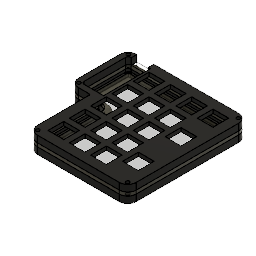
yampad_v2-Fusion360 (Autodesk Fusion 360 design; units mm, degrees)
Autodesk Fusion 360 part; units mm, degrees
(part 1 of 2)
sketch "PCB" plane through (0, 0, 0) normal (0, 1, 0) x (1, 0, 0) in component "MidLayer"
  line L0 (94.361, -93.472) -> (94.361, -1.778) construction
  arc A0 (-0.127, -38.608) -> (1.143, -39.878) centre (1.143, -38.608) ccw construction
  line L1 (92.583, 0) -> (1.397, 0) construction
  arc A1 (94.361, -1.778) -> (92.583, 0) centre (92.583, -1.778) ccw construction
  arc A2 (17.907, -93.218) -> (19.685, -94.996) centre (19.685, -93.218) ccw construction
  line L2 (17.907, -93.218) -> (17.907, -41.148) construction
  line L3 (19.685, -94.996) -> (92.837, -94.996) construction
  arc A3 (17.907, -41.148) -> (16.637, -39.878) centre (16.637, -41.148) ccw construction
  arc A4 (1.397, 0) -> (-0.127, -1.524) centre (1.397, -1.524) ccw construction
  line L4 (-0.127, -38.608) -> (-0.127, -1.524) construction
  arc A5 (92.837, -94.996) -> (94.361, -93.472) centre (92.837, -93.472) ccw construction
  line L5 (16.637, -39.878) -> (1.143, -39.878) construction
  line L6 (16.637, -39.878) -> (1.143, -39.878) construction
  line L7 (77.978, -44.958) -> (77.978, -30.988) construction
  line L8 (-0.127, -38.608) -> (-0.127, -1.524) construction
  arc A6 (92.837, -94.996) -> (94.361, -93.472) centre (92.837, -93.472) ccw construction
  arc A7 (94.361, -1.778) -> (92.583, 0) centre (92.583, -1.778) ccw construction
  line L9 (91.948, -30.988) -> (91.948, -44.958) construction
  line L10 (5.334, -3.81) -> (5.334, 1.524) construction
  line L11 (94.361, -93.472) -> (94.361, -1.778) construction
  line L12 (39.878, -16.383) -> (39.878, -2.413) construction
  line L13 (12.954, 1.524) -> (12.954, -3.81) construction
  line L14 (58.928, -2.413) -> (72.898, -2.413) construction
  line L15 (91.948, -44.958) -> (77.978, -44.958) construction
  line L16 (72.898, -40.513) -> (72.898, -54.483) construction
  line L17 (77.978, -2.413) -> (91.948, -2.413) construction
  line L18 (77.978, -69.088) -> (91.948, -69.088) construction
  line L19 (58.928, -21.463) -> (72.898, -21.463) construction
  line L20 (39.878, -21.463) -> (53.848, -21.463) construction
  line L21 (72.898, -21.463) -> (72.898, -35.433) construction
  line L22 (17.907, -93.218) -> (17.907, -41.148) construction
  arc A8 (1.397, 0) -> (-0.127, -1.524) centre (1.397, -1.524) ccw construction
  arc A9 (17.907, -41.148) -> (16.637, -39.878) centre (16.637, -41.148) ccw construction
  line L23 (12.954, -3.81) -> (5.334, -3.81) construction
  line L24 (39.878, -2.413) -> (53.848, -2.413) construction
  line L25 (72.898, -35.433) -> (58.928, -35.433) construction
  line L26 (39.878, -35.433) -> (39.878, -21.463) construction
  line L27 (58.928, -16.383) -> (58.928, -2.413) construction
  line L28 (72.898, -16.383) -> (58.928, -16.383) construction
  line L29 (20.828, -40.513) -> (34.798, -40.513) construction
  line L30 (91.948, -2.413) -> (91.948, -16.383) construction
  line L31 (91.948, -16.383) -> (77.978, -16.383) construction
  line L32 (53.848, -21.463) -> (53.848, -35.433) construction
  line L33 (77.978, -83.058) -> (77.978, -69.088) construction
  line L34 (53.848, -16.383) -> (39.878, -16.383) construction
  line L35 (72.898, -54.483) -> (58.928, -54.483) construction
  line L36 (58.928, -40.513) -> (72.898, -40.513) construction
  line L37 (77.978, -30.988) -> (91.948, -30.988) construction
  line L38 (91.948, -83.058) -> (77.978, -83.058) construction
  arc A10 (-0.127, -38.608) -> (1.143, -39.878) centre (1.143, -38.608) ccw construction
  line L39 (0, -39.878) -> (0, 0) construction
  arc A11 (17.907, -93.218) -> (19.685, -94.996) centre (19.685, -93.218) ccw construction
  line L40 (91.948, -69.088) -> (91.948, -83.058) construction
  line L41 (0, 0) -> (18.161, 0) construction
  line L42 (18.161, -39.878) -> (0, -39.878) construction
  line L43 (5.334, 1.524) -> (12.954, 1.524) construction
  line L44 (18.161, 0) -> (18.161, -39.878) construction
  line L45 (20.828, -35.433) -> (20.828, -21.463) construction
  line L46 (92.583, 0) -> (1.397, 0) construction
  line L47 (19.685, -94.996) -> (92.837, -94.996) construction
  line L48 (34.798, -35.433) -> (20.828, -35.433) construction
  line L49 (72.898, -59.563) -> (72.898, -73.533) construction
  line L50 (34.798, -73.533) -> (20.828, -73.533) construction
  line L51 (34.798, -92.583) -> (20.828, -92.583) construction
  line L52 (39.878, -54.483) -> (39.878, -40.513) construction
  line L53 (53.848, -78.613) -> (53.848, -92.583) construction
  line L54 (58.928, -73.533) -> (58.928, -59.563) construction
  line L55 (39.878, -78.613) -> (53.848, -78.613) construction
  line L56 (53.848, -92.583) -> (39.878, -92.583) construction
  line L57 (20.828, -21.463) -> (34.798, -21.463) construction
  line L58 (34.798, -78.613) -> (34.798, -92.583) construction
  line L59 (58.928, -59.563) -> (72.898, -59.563) construction
  line L60 (34.798, -21.463) -> (34.798, -35.433) construction
  line L61 (34.798, -16.383) -> (20.828, -16.383) construction
  line L62 (53.848, -59.563) -> (53.848, -73.533) construction
  line L63 (20.828, -54.483) -> (20.828, -40.513) construction
  line L64 (39.878, -40.513) -> (53.848, -40.513) construction
  line L65 (39.878, -73.533) -> (39.878, -59.563) construction
  line L66 (53.848, -73.533) -> (39.878, -73.533) construction
  line L67 (53.848, -40.513) -> (53.848, -54.483) construction
  line L68 (72.898, -73.533) -> (58.928, -73.533) construction
  line L69 (20.828, -78.613) -> (34.798, -78.613) construction
  line L70 (58.928, -35.433) -> (58.928, -21.463) construction
  line L71 (39.878, -92.583) -> (39.878, -78.613) construction
  line L72 (20.828, -92.583) -> (20.828, -78.613) construction
  line L73 (34.798, -59.563) -> (34.798, -73.533) construction
  line L74 (58.928, -92.583) -> (58.928, -78.613) construction
  line L75 (53.848, -54.483) -> (39.878, -54.483) construction
  line L76 (77.978, -16.383) -> (77.978, -2.413) construction
  line L77 (72.898, -92.583) -> (58.928, -92.583) construction
  line L78 (20.828, -59.563) -> (34.798, -59.563) construction
  line L79 (58.928, -78.613) -> (72.898, -78.613) construction
  line L80 (20.828, -16.383) -> (20.828, -2.413) construction
  line L81 (20.828, -73.533) -> (20.828, -59.563) construction
  line L82 (53.848, -35.433) -> (39.878, -35.433) construction
  line L83 (58.928, -54.483) -> (58.928, -40.513) construction
  line L84 (53.848, -2.413) -> (53.848, -16.383) construction
  line L85 (72.898, -78.613) -> (72.898, -92.583) construction
  line L86 (34.798, -2.413) -> (34.798, -16.383) construction
  line L87 (34.798, -54.483) -> (20.828, -54.483) construction
  line L88 (34.798, -40.513) -> (34.798, -54.483) construction
  line L89 (20.828, -2.413) -> (34.798, -2.413) construction
  line L90 (39.878, -59.563) -> (53.848, -59.563) construction
  line L91 (72.898, -2.413) -> (72.898, -16.383) construction
  line L92 (95.361, -93.472) -> (95.361, -1.778)
  arc A12 (95.361, -1.778) -> (92.583, 1) centre (92.583, -1.778) ccw
  line L93 (92.583, 1) -> (1.397, 1)
  arc A13 (1.397, 1) -> (-1.127, -1.524) centre (1.397, -1.524) ccw
  line L94 (-1.127, -38.608) -> (-1.127, -1.524)
  arc A14 (-1.127, -38.608) -> (1.143, -40.878) centre (1.143, -38.608) ccw
  line L95 (16.637, -40.878) -> (1.143, -40.878) construction
  arc A15 (16.907, -41.148) -> (16.637, -40.878) centre (16.637, -41.148) ccw construction
  line L96 (16.907, -93.218) -> (16.907, -41.148) construction
  arc A16 (16.907, -93.218) -> (19.685, -95.996) centre (19.685, -93.218) ccw
  line L97 (19.685, -95.996) -> (92.837, -95.996)
  arc A17 (92.837, -95.996) -> (95.361, -93.472) centre (92.837, -93.472) ccw
  line L98 (100.361, -93.472) -> (100.361, -1.778)
  arc A18 (100.361, -1.778) -> (92.583, 6) centre (92.583, -1.778) ccw
  line L99 (92.583, 6) -> (1.397, 6)
  arc A19 (1.397, 6) -> (-6.127, -1.524) centre (1.397, -1.524) ccw
  line L100 (-6.127, -38.608) -> (-6.127, -1.524)
  arc A20 (-6.127, -38.608) -> (1.143, -45.878) centre (1.143, -38.608) ccw
  line L101 (11.907, -45.878) -> (1.143, -45.878) construction
  line L102 (11.907, -93.218) -> (11.907, -45.878) construction
  arc A21 (11.907, -93.218) -> (19.685, -100.996) centre (19.685, -93.218) ccw
  line L103 (19.685, -100.996) -> (92.837, -100.996)
  arc A22 (92.837, -100.996) -> (100.361, -93.472) centre (92.837, -93.472) ccw
  line L104 (1.143, -40.878) -> (13.907, -40.878)
  line L105 (16.907, -93.218) -> (16.907, -43.878)
  arc A23 (16.907, -43.878) -> (13.907, -40.878) centre (13.907, -43.878) ccw
  line L106 (1.143, -45.878) -> (10.907, -45.878)
  line L107 (11.907, -46.878) -> (11.907, -93.218)
  arc A24 (11.907, -46.878) -> (10.907, -45.878) centre (10.907, -46.878) ccw
  dimension "d7" = 1
  dimension "d8" = 6
  dimension "d10" = 3
  dimension "d11" = 1
  constraint tangent A14 L104
  constraint perpendicular L96 L104
  constraint tangent A16 L105
  constraint tangent L104 A23
  constraint tangent L105 A23
  constraint tangent A20 L106
  constraint tangent A21 L107
  constraint coincident L101.start L107
  constraint coincident L101.start L106
  constraint tangent L107 A24
  constraint tangent L106 A24
  measures "d10" radius of A23
  measures "d11" radius of A24
extrude "Extrude1" add sketch "PCB" along normal blind 3 makes body 1 in component "MidLayer"
sketch "Sketch1" plane through (0, 3, 0) normal (0, 1, 0) x (-1, 0, 0) in component "TopLayer"
  arc A0 (-16.907, 93.218) -> (-19.685, 95.996) centre (-19.685, 93.218) ccw construction
  line L0 (-16.907, 93.218) -> (-16.907, 43.878) construction
  arc A1 (-16.907, 43.878) -> (-13.907, 40.878) centre (-13.907, 43.878) ccw construction
  line L1 (-13.907, 40.878) -> (-1.143, 40.878)
  arc A2 (1.127, 38.608) -> (-1.143, 40.878) centre (-1.143, 38.608) ccw
  line L2 (1.127, 38.608) -> (1.127, 1.524)
  arc A3 (-1.397, -1) -> (1.127, 1.524) centre (-1.397, 1.524) ccw
  line L3 (-1.397, -1) -> (-92.583, -1) construction
  arc A4 (-95.361, 1.778) -> (-92.583, -1) centre (-92.583, 1.778) ccw construction
  line L4 (-95.361, 1.778) -> (-95.361, 93.472) construction
  arc A5 (-92.837, 95.996) -> (-95.361, 93.472) centre (-92.837, 93.472) ccw construction
  line L5 (-92.837, 95.996) -> (-19.685, 95.996) construction
  arc A6 (-11.907, 93.218) -> (-19.685, 100.996) centre (-19.685, 93.218) ccw
  line L6 (-19.685, 100.996) -> (-92.837, 100.996)
  arc A7 (-92.837, 100.996) -> (-100.361, 93.472) centre (-92.837, 93.472) ccw
  line L7 (-100.361, 93.472) -> (-100.361, 1.778)
  arc A8 (-100.361, 1.778) -> (-92.583, -6) centre (-92.583, 1.778) ccw
  line L8 (-92.583, -6) -> (-1.397, -6)
  arc A9 (-1.397, -6) -> (6.127, 1.524) centre (-1.397, 1.524) ccw
  line L9 (6.127, 1.524) -> (6.127, 38.608)
  arc A10 (6.127, 38.608) -> (-1.143, 45.878) centre (-1.143, 38.608) ccw
  line L10 (-1.143, 45.878) -> (-10.907, 45.878)
  arc A11 (-11.907, 46.878) -> (-10.907, 45.878) centre (-10.907, 46.878) ccw
  line L11 (-11.907, 46.878) -> (-11.907, 93.218)
  line L12 (-20.828, 2.413) -> (-34.798, 16.383) construction
  line L13 (-39.878, 2.413) -> (-53.848, 16.383) construction
  line L14 (-58.928, 2.413) -> (-72.898, 16.383) construction
  line L15 (-77.978, 2.413) -> (-91.948, 16.383) construction
  line L16 (-20.828, 21.463) -> (-34.798, 35.433) construction
  line L17 (-39.878, 21.463) -> (-53.848, 35.433) construction
  line L18 (-58.928, 21.463) -> (-72.898, 35.433) construction
  line L19 (-77.978, 30.988) -> (-91.948, 44.958) construction
  line L20 (-20.828, 40.513) -> (-34.798, 54.483) construction
  line L21 (-39.878, 40.513) -> (-53.848, 54.483) construction
  line L22 (-58.928, 40.513) -> (-72.898, 54.483) construction
  line L23 (-20.828, 59.563) -> (-34.798, 73.533) construction
  line L24 (-39.878, 59.563) -> (-53.848, 73.533) construction
  line L25 (-58.928, 59.563) -> (-72.898, 73.533) construction
  line L26 (-77.978, 69.088) -> (-91.948, 83.058) construction
  line L27 (-20.828, 78.613) -> (-34.798, 92.583) construction
  line L28 (-39.878, 78.613) -> (-53.848, 92.583) construction
  line L29 (-58.928, 78.613) -> (-72.898, 92.583) construction
  line L30 (-34.838, 16.423) -> (-20.788, 16.423)
  line L31 (-20.788, 16.423) -> (-20.788, 2.373)
  line L32 (-20.788, 2.373) -> (-34.838, 2.373)
  line L33 (-34.838, 2.373) -> (-34.838, 16.423)
  line L34 (-34.838, 16.423) -> (-20.788, 2.373) construction
  line L35 (-20.788, 16.423) -> (-34.838, 2.373) construction
  line L36 (-53.888, 16.423) -> (-39.838, 16.423)
  line L37 (-39.838, 16.423) -> (-39.838, 2.373)
  line L38 (-39.838, 2.373) -> (-53.888, 2.373)
  line L39 (-53.888, 2.373) -> (-53.888, 16.423)
  line L40 (-53.888, 16.423) -> (-39.838, 2.373) construction
  line L41 (-39.838, 16.423) -> (-53.888, 2.373) construction
  line L42 (-34.838, 35.473) -> (-20.788, 35.473)
  line L43 (-20.788, 35.473) -> (-20.788, 21.423)
  line L44 (-20.788, 21.423) -> (-34.838, 21.423)
  line L45 (-34.838, 21.423) -> (-34.838, 35.473)
  line L46 (-34.838, 35.473) -> (-20.788, 21.423) construction
  line L47 (-20.788, 35.473) -> (-34.838, 21.423) construction
  line L48 (-72.938, 16.423) -> (-58.888, 16.423)
  line L49 (-58.888, 16.423) -> (-58.888, 2.373)
  line L50 (-58.888, 2.373) -> (-72.938, 2.373)
  line L51 (-72.938, 2.373) -> (-72.938, 16.423)
  line L52 (-72.938, 16.423) -> (-58.888, 2.373) construction
  line L53 (-58.888, 16.423) -> (-72.938, 2.373) construction
  line L54 (-91.988, 16.423) -> (-77.938, 16.423)
  line L55 (-77.938, 16.423) -> (-77.938, 2.373)
  line L56 (-77.938, 2.373) -> (-91.988, 2.373)
  line L57 (-91.988, 2.373) -> (-91.988, 16.423)
  line L58 (-91.988, 16.423) -> (-77.938, 2.373) construction
  line L59 (-77.938, 16.423) -> (-91.988, 2.373) construction
  line L60 (-53.888, 35.473) -> (-39.838, 35.473)
  line L61 (-39.838, 35.473) -> (-39.838, 21.423)
  line L62 (-39.838, 21.423) -> (-53.888, 21.423)
  line L63 (-53.888, 21.423) -> (-53.888, 35.473)
  line L64 (-53.888, 35.473) -> (-39.838, 21.423) construction
  line L65 (-39.838, 35.473) -> (-53.888, 21.423) construction
  line L66 (-72.938, 35.473) -> (-58.888, 35.473)
  line L67 (-58.888, 35.473) -> (-58.888, 21.423)
  line L68 (-58.888, 21.423) -> (-72.938, 21.423)
  line L69 (-72.938, 21.423) -> (-72.938, 35.473)
  line L70 (-72.938, 35.473) -> (-58.888, 21.423) construction
  line L71 (-58.888, 35.473) -> (-72.938, 21.423) construction
  line L72 (-91.988, 44.998) -> (-77.938, 44.998)
  line L73 (-77.938, 44.998) -> (-77.938, 30.948)
  line L74 (-77.938, 30.948) -> (-91.988, 30.948)
  line L75 (-91.988, 30.948) -> (-91.988, 44.998)
  line L76 (-91.988, 44.998) -> (-77.938, 30.948) construction
  line L77 (-77.938, 44.998) -> (-91.988, 30.948) construction
  line L78 (-72.938, 54.523) -> (-58.888, 54.523)
  line L79 (-58.888, 54.523) -> (-58.888, 40.473)
  line L80 (-58.888, 40.473) -> (-72.938, 40.473)
  line L81 (-72.938, 40.473) -> (-72.938, 54.523)
  line L82 (-72.938, 54.523) -> (-58.888, 40.473) construction
  line L83 (-58.888, 54.523) -> (-72.938, 40.473) construction
  line L84 (-53.888, 54.523) -> (-39.838, 54.523)
  line L85 (-39.838, 54.523) -> (-39.838, 40.473)
  line L86 (-39.838, 40.473) -> (-53.888, 40.473)
  line L87 (-53.888, 40.473) -> (-53.888, 54.523)
  line L88 (-53.888, 54.523) -> (-39.838, 40.473) construction
  line L89 (-39.838, 54.523) -> (-53.888, 40.473) construction
  line L90 (-34.838, 54.523) -> (-20.788, 54.523)
  line L91 (-20.788, 54.523) -> (-20.788, 40.473)
  line L92 (-20.788, 40.473) -> (-34.838, 40.473)
  line L93 (-34.838, 40.473) -> (-34.838, 54.523)
  line L94 (-34.838, 54.523) -> (-20.788, 40.473) construction
  line L95 (-20.788, 54.523) -> (-34.838, 40.473) construction
  line L96 (-34.838, 73.573) -> (-20.788, 73.573)
  line L97 (-20.788, 73.573) -> (-20.788, 59.523)
  line L98 (-20.788, 59.523) -> (-34.838, 59.523)
  line L99 (-34.838, 59.523) -> (-34.838, 73.573)
  line L100 (-34.838, 73.573) -> (-20.788, 59.523) construction
  line L101 (-20.788, 73.573) -> (-34.838, 59.523) construction
  line L102 (-53.888, 73.573) -> (-39.838, 73.573)
  line L103 (-39.838, 73.573) -> (-39.838, 59.523)
  line L104 (-39.838, 59.523) -> (-53.888, 59.523)
  line L105 (-53.888, 59.523) -> (-53.888, 73.573)
  line L106 (-53.888, 73.573) -> (-39.838, 59.523) construction
  line L107 (-39.838, 73.573) -> (-53.888, 59.523) construction
  line L108 (-72.938, 73.573) -> (-58.888, 73.573)
  line L109 (-58.888, 73.573) -> (-58.888, 59.523)
  line L110 (-58.888, 59.523) -> (-72.938, 59.523)
  line L111 (-72.938, 59.523) -> (-72.938, 73.573)
  line L112 (-72.938, 73.573) -> (-58.888, 59.523) construction
  line L113 (-58.888, 73.573) -> (-72.938, 59.523) construction
  line L114 (-91.988, 83.098) -> (-77.938, 83.098)
  line L115 (-77.938, 83.098) -> (-77.938, 69.048)
  line L116 (-77.938, 69.048) -> (-91.988, 69.048)
  line L117 (-91.988, 69.048) -> (-91.988, 83.098)
  line L118 (-91.988, 83.098) -> (-77.938, 69.048) construction
  line L119 (-77.938, 83.098) -> (-91.988, 69.048) construction
  line L120 (-72.938, 92.623) -> (-58.888, 92.623)
  line L121 (-58.888, 92.623) -> (-58.888, 78.573)
  line L122 (-58.888, 78.573) -> (-72.938, 78.573)
  line L123 (-72.938, 78.573) -> (-72.938, 92.623)
  line L124 (-72.938, 92.623) -> (-58.888, 78.573) construction
  line L125 (-58.888, 92.623) -> (-72.938, 78.573) construction
  line L126 (-53.888, 92.623) -> (-39.838, 92.623)
  line L127 (-39.838, 92.623) -> (-39.838, 78.573)
  line L128 (-39.838, 78.573) -> (-53.888, 78.573)
  line L129 (-53.888, 78.573) -> (-53.888, 92.623)
  line L130 (-53.888, 92.623) -> (-39.838, 78.573) construction
  line L131 (-39.838, 92.623) -> (-53.888, 78.573) construction
  line L132 (-34.838, 92.623) -> (-20.788, 92.623)
  line L133 (-20.788, 92.623) -> (-20.788, 78.573)
  line L134 (-20.788, 78.573) -> (-34.838, 78.573)
  line L135 (-34.838, 78.573) -> (-34.838, 92.623)
  line L136 (-34.838, 92.623) -> (-20.788, 78.573) construction
  line L137 (-20.788, 92.623) -> (-34.838, 78.573) construction
  line L138 (-18.161, 0) -> (0, 0) construction
  line L139 (0, 0) -> (0, 39.878) construction
  line L140 (0, 39.878) -> (-18.161, 39.878) construction
  line L141 (-18.161, 39.878) -> (-18.161, 0) construction
  line L142 (-16.644, -6) -> (-1.644, -6)
  line L143 (0.5, -0.5) -> (0.5, 40.378) construction
  line L144 (0.5, 40.378) -> (-18.661, 40.378) construction
  line L145 (-18.661, 40.378) -> (-18.661, -0.5)
  line L146 (-18.661, -0.5) -> (0.5, -0.5) construction
  line L147 (-18.661, -0.5) -> (-18.661, -1)
  line L148 (-18.661, -1) -> (-1.397, -1)
  line L149 (-13.907, 40.878) -> (-18.661, 40.878)
  line L150 (-18.661, 40.878) -> (-18.661, 40.378)
  line L151 (-12.954, -0.5) -> (-12.954, -6) construction
  line L152 (-92.583, -6) -> (-1.397, -6)
  line L153 (-12.954, -6) -> (-5.334, -0.5) construction
  line L154 (-1.644, -6) -> (-16.644, -6)
  line L155 (-16.644, -6) -> (-16.644, -0.5)
  line L156 (-16.644, -0.5) -> (-1.644, -0.5)
  line L157 (-1.644, -0.5) -> (-1.644, -6)
  line L158 (-1.644, -6) -> (-16.644, -0.5) construction
  line L159 (-16.644, -6) -> (-1.644, -0.5) construction
  point P0 (-20.828, 2.413)
  point P1 (-34.798, 16.383)
  point P2 (-39.878, 2.413)
  point P3 (-53.848, 16.383)
  point P4 (-58.928, 2.413)
  point P5 (-72.898, 16.383)
  point P6 (-77.978, 2.413)
  point P7 (-91.948, 16.383)
  point P8 (-20.828, 21.463)
  point P9 (-34.798, 35.433)
  point P10 (-39.878, 21.463)
  point P11 (-53.848, 35.433)
  point P12 (-58.928, 21.463)
  point P13 (-72.898, 35.433)
  point P14 (-77.978, 30.988)
  point P15 (-91.948, 44.958)
  point P16 (-20.828, 40.513)
  point P17 (-34.798, 54.483)
  point P18 (-39.878, 40.513)
  point P19 (-53.848, 54.483)
  point P20 (-58.928, 40.513)
  point P21 (-72.898, 54.483)
  point P22 (-20.828, 59.563)
  point P23 (-34.798, 73.533)
  point P24 (-39.878, 59.563)
  point P25 (-53.848, 73.533)
  point P26 (-58.928, 59.563)
  point P27 (-72.898, 73.533)
  point P28 (-77.978, 69.088)
  point P29 (-91.948, 83.058)
  point P30 (-20.828, 78.613)
  point P31 (-34.798, 92.583)
  point P32 (-39.878, 78.613)
  point P33 (-53.848, 92.583)
  point P34 (-58.928, 78.613)
  point P35 (-72.898, 92.583)
  point P36 (-27.813, 9.398)
  point P37 (-46.863, 9.398)
  point P38 (-27.813, 28.448)
  point P39 (-65.913, 9.398)
  point P40 (-84.963, 9.398)
  point P41 (-46.863, 28.448)
  point P42 (-65.913, 28.448)
  point P43 (-84.963, 37.973)
  point P44 (-65.913, 47.498)
  point P45 (-46.863, 47.498)
  point P46 (-27.813, 47.498)
  point P47 (-27.813, 66.548)
  point P48 (-46.863, 66.548)
  point P49 (-65.913, 66.548)
  point P50 (-84.963, 76.073)
  point P51 (-65.913, 85.598)
  point P52 (-46.863, 85.598)
  point P53 (-27.813, 85.598)
  point P54 (-18.161, 0)
  point P55 (0, 39.878)
  point P56 (-5.334, -0.5)
  point P57 (-12.954, -0.5)
  point P58 (-9.144, -3.25)
  dimension "d14" = 14.05
  dimension "d15" = 14.05
  dimension "d16" = 14.05
  dimension "d17" = 14.05
  dimension "d18" = 14.05
  dimension "d19" = 14.05
  dimension "d20" = 14.05
  dimension "d21" = 14.05
  dimension "d26" = 0.5
  dimension "d27" = 15
  constraint coincident P0 L12.start
  constraint coincident P1 L12.end
  constraint coincident P2 L13.start
  constraint coincident P3 L13.end
  constraint coincident P4 L14.start
  constraint coincident P5 L14.end
  constraint coincident P6 L15.start
  constraint coincident P7 L15.end
  constraint coincident P8 L16.start
  constraint coincident P9 L16.end
  constraint coincident P10 L17.start
  constraint coincident P11 L17.end
  constraint coincident P12 L18.start
  constraint coincident P13 L18.end
  constraint coincident P14 L19.start
  constraint coincident P15 L19.end
  constraint coincident P16 L20.start
  constraint coincident P17 L20.end
  constraint coincident P18 L21.start
  constraint coincident P19 L21.end
  constraint coincident P20 L22.start
  constraint coincident P21 L22.end
  constraint coincident P22 L23.start
  constraint coincident P23 L23.end
  constraint coincident P24 L24.start
  constraint coincident P25 L24.end
  constraint coincident P26 L25.start
  constraint coincident P27 L25.end
  constraint coincident P28 L26.start
  constraint coincident P29 L26.end
  constraint coincident P30 L27.start
  constraint coincident P31 L27.end
  constraint coincident P32 L28.start
  constraint coincident P33 L28.end
  constraint coincident P34 L29.start
  constraint coincident P35 L29.end
  constraint perpendicular L30 L31
  constraint parallel L30 L32
  constraint parallel L31 L33
  constraint horizontal L30
  constraint coincident L34 P36
  constraint coincident L35 P36
  constraint midpoint L12 P36
  constraint perpendicular L36 L37
  constraint parallel L36 L38
  constraint parallel L37 L39
  constraint horizontal L36
  constraint coincident L40 P37
  constraint coincident L41 P37
  constraint midpoint L13 P37
  constraint perpendicular L42 L43
  constraint parallel L42 L44
  constraint parallel L43 L45
  constraint horizontal L42
  constraint coincident L46 P38
  constraint coincident L47 P38
  constraint midpoint L16 P38
  constraint perpendicular L48 L49
  constraint parallel L48 L50
  constraint parallel L49 L51
  constraint horizontal L48
  constraint coincident L52 P39
  constraint coincident L53 P39
  constraint midpoint L14 P39
  constraint perpendicular L54 L55
  constraint parallel L54 L56
  constraint parallel L55 L57
  constraint horizontal L54
  constraint coincident L15 L54.start
  constraint coincident L58 P40
  constraint coincident L59 P40
  constraint midpoint L15 P40
  constraint equal L50 L56
  constraint perpendicular L60 L61
  constraint parallel L60 L62
  constraint parallel L61 L63
  constraint horizontal L60
  constraint coincident L17 L60.start
  constraint coincident L64 P41
  constraint coincident L65 P41
  constraint midpoint L17 P41
  constraint perpendicular L66 L67
  constraint parallel L66 L68
  constraint parallel L67 L69
  constraint horizontal L66
  constraint coincident L18 L66.start
  constraint coincident L70 P42
  constraint coincident L71 P42
  constraint midpoint L18 P42
  constraint perpendicular L72 L73
  constraint parallel L72 L74
  constraint parallel L73 L75
  constraint horizontal L72
  constraint coincident L19 L72.start
  constraint coincident L76 P43
  constraint coincident L77 P43
  constraint midpoint L19 P43
  constraint perpendicular L78 L79
  constraint parallel L78 L80
  constraint parallel L79 L81
  constraint horizontal L78
  constraint coincident L22 L78.start
  constraint coincident L82 P44
  constraint coincident L83 P44
  constraint midpoint L22 P44
  constraint perpendicular L84 L85
  constraint parallel L84 L86
  constraint parallel L85 L87
  constraint horizontal L84
  constraint coincident L21 L84.start
  constraint coincident L88 P45
  constraint coincident L89 P45
  constraint midpoint L21 P45
  constraint perpendicular L90 L91
  constraint parallel L90 L92
  constraint parallel L91 L93
  constraint horizontal L90
  constraint coincident L20 L90.start
  constraint coincident L94 P46
  constraint coincident L95 P46
  constraint midpoint L20 P46
  constraint equal L86 L92
  constraint equal L80 L86
  constraint equal L74 L80
  constraint equal L68 L74
  constraint equal L62 L68
  constraint equal L44 L62
  constraint perpendicular L96 L97
  constraint parallel L96 L98
  constraint parallel L97 L99
  constraint horizontal L96
  constraint coincident L23 L96.start
  constraint coincident L100 P47
  constraint coincident L101 P47
  constraint midpoint L23 P47
  constraint perpendicular L102 L103
  constraint parallel L102 L104
  constraint parallel L103 L105
  constraint horizontal L102
  constraint coincident L24 L102.start
  constraint coincident L106 P48
  constraint coincident L107 P48
  constraint midpoint L24 P48
  constraint perpendicular L108 L109
  constraint parallel L108 L110
  constraint parallel L109 L111
  constraint horizontal L108
  constraint coincident L25 L108.start
  constraint coincident L112 P49
  constraint coincident L113 P49
  constraint midpoint L25 P49
  constraint perpendicular L114 L115
  constraint parallel L114 L116
  constraint parallel L115 L117
  constraint horizontal L114
  constraint coincident L26 L114.start
  constraint coincident L118 P50
  constraint coincident L119 P50
  constraint midpoint L26 P50
  constraint perpendicular L120 L121
  constraint parallel L120 L122
  constraint parallel L121 L123
  constraint horizontal L120
  constraint coincident L29 L120.start
  constraint coincident L124 P51
  constraint coincident L125 P51
  constraint midpoint L29 P51
  constraint perpendicular L126 L127
  constraint parallel L126 L128
  constraint parallel L127 L129
  constraint horizontal L126
  constraint coincident L28 L126.start
  constraint coincident L130 P52
  constraint coincident L131 P52
  constraint midpoint L28 P52
  constraint perpendicular L132 L133
  constraint parallel L132 L134
  constraint parallel L133 L135
  constraint horizontal L132
  constraint coincident L27 L132.start
  constraint coincident L136 P53
  constraint coincident L137 P53
  constraint midpoint L27 P53
  constraint equal L98 L104
  constraint equal L104 L110
  constraint equal L110 L116
  constraint equal L116 L122
  constraint equal L122 L128
  constraint equal L128 L134
  constraint equal L72 L134
  constraint horizontal L138
  constraint vertical L139
  constraint horizontal L140
  constraint vertical L141
  constraint coincident P55 L139.end
  constraint coincident P54 L138.start
  constraint horizontal L142
  constraint coincident L3 L147.end
  constraint perpendicular L3 L147
  constraint coincident A3.start L3.start
  constraint coincident A1.end L1.start
  constraint tangent A1 L149
  constraint perpendicular L145 L149
  constraint perpendicular L144 L150
  constraint coincident P57 L151.start
  constraint perpendicular L146 L151
  constraint coincident L151.end L152
  constraint coincident P56 L153.end
  constraint perpendicular L154 L155
  constraint parallel L154 L156
  constraint parallel L155 L157
  constraint horizontal L154
  constraint coincident L158 P58
  constraint coincident L159 P58
  constraint midpoint L153 P58
  measures "d14" distance of L31.end L32.end
  measures "d15" distance of L30.end L31.end
  measures "d16" distance of L37.end L38.end
  measures "d17" distance of L36.end L37.end
  measures "d18" distance of L43.end L44.end
  measures "d19" distance of L42.end L43.end
  measures "d20" distance of L48.end L49.end
  measures "d21" distance of L49.end L50.end
  measures "d27" distance of L155.end L156.end
extrude "Extrude1'" add sketch "Sketch1" along normal blind 6 separate body contours L1 A2 L2 A3 A6 L6 A7 L7 A8 L8 A9 L9 A10 L10 A11 L11 L145 L147 L148 L149 L150 L152 L155 L157 makes body 2 in component "TopLayer"
sketch "Sketch2" plane through (0, 3, 0) normal (0, -1, 0) x (1, 0, 0) in component "TopLayer"
  line L0 (91.988, 2.373) -> (77.938, 2.373)
  line L1 (77.938, 2.373) -> (77.938, 16.423)
  line L2 (77.938, 16.423) -> (91.988, 16.423)
  line L3 (91.988, 16.423) -> (91.988, 2.373)
  line L4 (72.938, 2.373) -> (58.888, 2.373)
  line L5 (58.888, 2.373) -> (58.888, 16.423)
  line L6 (58.888, 16.423) -> (72.938, 16.423)
  line L7 (72.938, 16.423) -> (72.938, 2.373)
  line L8 (34.838, 2.373) -> (20.788, 2.373)
  line L9 (20.788, 2.373) -> (20.788, 16.423)
  line L10 (20.788, 16.423) -> (34.838, 16.423)
  line L11 (34.838, 16.423) -> (34.838, 2.373)
  line L12 (53.888, 2.373) -> (39.838, 2.373)
  line L13 (39.838, 2.373) -> (39.838, 16.423)
  line L14 (39.838, 16.423) -> (53.888, 16.423)
  line L15 (53.888, 16.423) -> (53.888, 2.373)
  line L16 (53.888, 59.523) -> (39.838, 59.523)
  line L17 (39.838, 59.523) -> (39.838, 73.573)
  line L18 (39.838, 73.573) -> (53.888, 73.573)
  line L19 (53.888, 73.573) -> (53.888, 59.523)
  line L20 (72.938, 21.423) -> (58.888, 21.423)
  line L21 (58.888, 21.423) -> (58.888, 35.473)
  line L22 (58.888, 35.473) -> (72.938, 35.473)
  line L23 (72.938, 35.473) -> (72.938, 21.423)
  line L24 (34.838, 78.573) -> (20.788, 78.573)
  line L25 (20.788, 78.573) -> (20.788, 92.623)
  line L26 (20.788, 92.623) -> (34.838, 92.623)
  line L27 (34.838, 92.623) -> (34.838, 78.573)
  line L28 (34.838, 40.473) -> (20.788, 40.473)
  line L29 (20.788, 40.473) -> (20.788, 54.523)
  line L30 (20.788, 54.523) -> (34.838, 54.523)
  line L31 (34.838, 54.523) -> (34.838, 40.473)
  line L32 (34.838, 59.523) -> (20.788, 59.523)
  line L33 (20.788, 59.523) -> (20.788, 73.573)
  line L34 (20.788, 73.573) -> (34.838, 73.573)
  line L35 (34.838, 73.573) -> (34.838, 59.523)
  line L36 (72.938, 59.523) -> (58.888, 59.523)
  line L37 (58.888, 59.523) -> (58.888, 73.573)
  line L38 (58.888, 73.573) -> (72.938, 73.573)
  line L39 (72.938, 73.573) -> (72.938, 59.523)
  line L40 (91.988, 30.948) -> (77.938, 30.948)
  line L41 (77.938, 30.948) -> (77.938, 44.998)
  line L42 (77.938, 44.998) -> (91.988, 44.998)
  line L43 (91.988, 44.998) -> (91.988, 30.948)
  line L44 (72.938, 40.473) -> (58.888, 40.473)
  line L45 (58.888, 40.473) -> (58.888, 54.523)
  line L46 (58.888, 54.523) -> (72.938, 54.523)
  line L47 (72.938, 54.523) -> (72.938, 40.473)
  line L48 (72.938, 78.573) -> (58.888, 78.573)
  line L49 (58.888, 78.573) -> (58.888, 92.623)
  line L50 (58.888, 92.623) -> (72.938, 92.623)
  line L51 (72.938, 92.623) -> (72.938, 78.573)
  line L52 (53.888, 40.473) -> (39.838, 40.473)
  line L53 (39.838, 40.473) -> (39.838, 54.523)
  line L54 (39.838, 54.523) -> (53.888, 54.523)
  line L55 (53.888, 54.523) -> (53.888, 40.473)
  line L56 (53.888, 21.423) -> (39.838, 21.423)
  line L57 (39.838, 21.423) -> (39.838, 35.473)
  line L58 (39.838, 35.473) -> (53.888, 35.473)
  line L59 (53.888, 35.473) -> (53.888, 21.423)
  line L60 (53.888, 78.573) -> (39.838, 78.573)
  line L61 (39.838, 78.573) -> (39.838, 92.623)
  line L62 (39.838, 92.623) -> (53.888, 92.623)
  line L63 (53.888, 92.623) -> (53.888, 78.573)
  line L64 (91.988, 69.048) -> (77.938, 69.048)
  line L65 (77.938, 69.048) -> (77.938, 83.098)
  line L66 (77.938, 83.098) -> (91.988, 83.098)
  line L67 (91.988, 83.098) -> (91.988, 69.048)
  line L68 (34.838, 21.423) -> (20.788, 21.423)
  line L69 (20.788, 21.423) -> (20.788, 35.473)
  line L70 (20.788, 35.473) -> (34.838, 35.473)
  line L71 (34.838, 35.473) -> (34.838, 21.423)
  line L72 (1.397, -6) -> (1.644, -6)
  arc A0 (92.583, -6) -> (100.361, 1.778) centre (92.583, 1.778) ccw
  line L73 (100.361, 1.778) -> (100.361, 93.472)
  arc A1 (100.361, 93.472) -> (92.837, 100.996) centre (92.837, 93.472) ccw
  line L74 (92.837, 100.996) -> (19.685, 100.996)
  arc A2 (19.685, 100.996) -> (11.907, 93.218) centre (19.685, 93.218) ccw
  line L75 (11.907, 93.218) -> (11.907, 46.878)
  arc A3 (10.907, 45.878) -> (11.907, 46.878) centre (10.907, 46.878) ccw
  line L76 (10.907, 45.878) -> (1.143, 45.878)
  arc A4 (1.143, 45.878) -> (-6.127, 38.608) centre (1.143, 38.608) ccw
  line L77 (-6.127, 38.608) -> (-6.127, 1.524)
  arc A5 (-6.127, 1.524) -> (1.397, -6) centre (1.397, 1.524) ccw
  line L78 (95.361, 93.472) -> (95.361, 1.778)
  arc A6 (92.583, -1) -> (95.361, 1.778) centre (92.583, 1.778) ccw
  line L79 (92.583, -1) -> (1.397, -1)
  arc A7 (-1.127, 1.524) -> (1.397, -1) centre (1.397, 1.524) ccw
  line L80 (-1.127, 38.608) -> (-1.127, 1.524)
  arc A8 (1.143, 40.878) -> (-1.127, 38.608) centre (1.143, 38.608) ccw
  line L81 (1.143, 40.878) -> (13.907, 40.878)
  arc A9 (13.907, 40.878) -> (16.907, 43.878) centre (13.907, 43.878) ccw
  line L82 (16.907, 93.218) -> (16.907, 43.878)
  arc A10 (19.685, 95.996) -> (16.907, 93.218) centre (19.685, 93.218) ccw
  line L83 (19.685, 95.996) -> (92.837, 95.996)
  arc A11 (95.361, 93.472) -> (92.837, 95.996) centre (92.837, 93.472) ccw
  line L84 (1.644, -6) -> (1.644, -1)
  line L85 (1.644, -1) -> (1.397, -1)
  arc A12 (-1.127, 1.524) -> (1.397, -1) centre (1.397, 1.524) ccw
  line L86 (-1.127, 1.524) -> (-1.127, 38.608)
  arc A13 (1.143, 40.878) -> (-1.127, 38.608) centre (1.143, 38.608) ccw
  line L87 (1.143, 40.878) -> (18.661, 40.878)
  line L88 (18.661, 40.878) -> (18.661, -1)
  line L89 (18.661, -1) -> (16.644, -1)
  line L90 (16.644, -1) -> (16.644, -6)
  line L91 (16.644, -6) -> (92.583, -6)
extrude "Extrude2" cut sketch "Sketch2" against normal blind 2.5 contours L78 A6 L79 A9 L82 A10 L83 A11 L87 L88 bodies 2 in component "TopLayer"
sketch "Sketch1 (2)" plane through (0, 0, 0) normal (0, 1, 0) x (1, 0, 0) in component "BaseLayer"
  line L0 (100.361, -93.472) -> (100.361, -1.778)
  arc A0 (16.907, -93.218) -> (19.685, -95.996) centre (19.685, -93.218) ccw construction
  line L1 (19.685, -95.996) -> (92.837, -95.996) construction
  arc A1 (92.837, -95.996) -> (95.361, -93.472) centre (92.837, -93.472) ccw construction
  line L2 (95.361, -93.472) -> (95.361, -1.778) construction
  arc A2 (95.361, -1.778) -> (92.583, 1) centre (92.583, -1.778) ccw construction
  line L3 (92.583, 1) -> (1.397, 1) construction
  arc A3 (1.397, 1) -> (-1.127, -1.524) centre (1.397, -1.524) ccw construction
  line L4 (-1.127, -1.524) -> (-1.127, -38.608) construction
  arc A4 (-1.127, -38.608) -> (1.143, -40.878) centre (1.143, -38.608) ccw construction
  line L5 (1.143, -40.878) -> (13.907, -40.878) construction
  arc A5 (16.907, -43.878) -> (13.907, -40.878) centre (13.907, -43.878) ccw construction
  line L6 (16.907, -43.878) -> (16.907, -93.218) construction
  arc A6 (11.907, -93.218) -> (19.685, -100.996) centre (19.685, -93.218) ccw
  line L7 (11.907, -93.218) -> (11.907, -46.878)
  arc A7 (11.907, -46.878) -> (10.907, -45.878) centre (10.907, -46.878) ccw
  line L8 (10.907, -45.878) -> (1.143, -45.878)
  arc A8 (-6.127, -38.608) -> (1.143, -45.878) centre (1.143, -38.608) ccw
  line L9 (-6.127, -38.608) -> (-6.127, -1.524)
  arc A9 (1.397, 6) -> (-6.127, -1.524) centre (1.397, -1.524) ccw
  line L10 (1.397, 6) -> (92.583, 6)
  arc A10 (100.361, -1.778) -> (92.583, 6) centre (92.583, -1.778) ccw
  line L11 (100.361, -1.778) -> (100.361, -93.472)
  arc A11 (92.837, -100.996) -> (100.361, -93.472) centre (92.837, -93.472) ccw
  line L12 (92.837, -100.996) -> (19.685, -100.996)
extrude "Extrude1''" add sketch "Sketch1 (2)" against normal blind 6 separate body makes body 3 in component "BaseLayer"
sketch "Sketch2 (2)" plane through (0, 0, 0) normal (0, 1, 0) x (-1, 0, 0) in component "BaseLayer"
  arc A0 (-100.361, 1.778) -> (-92.583, -6) centre (-92.583, 1.778) ccw
  line L0 (-92.583, -6) -> (-1.397, -6)
  arc A1 (-1.397, -6) -> (6.127, 1.524) centre (-1.397, 1.524) ccw
  line L1 (6.127, 1.524) -> (6.127, 38.608)
  arc A2 (6.127, 38.608) -> (-1.143, 45.878) centre (-1.143, 38.608) ccw
  line L2 (-1.143, 45.878) -> (-10.907, 45.878)
  arc A3 (-11.907, 46.878) -> (-10.907, 45.878) centre (-10.907, 46.878) ccw
  line L3 (-11.907, 46.878) -> (-11.907, 93.218)
  arc A4 (-11.907, 93.218) -> (-19.685, 100.996) centre (-19.685, 93.218) ccw
  line L4 (-19.685, 100.996) -> (-92.837, 100.996)
  arc A5 (-92.837, 100.996) -> (-100.361, 93.472) centre (-92.837, 93.472) ccw
  line L5 (-100.361, 93.472) -> (-100.361, 1.778)
  arc A6 (-16.907, 93.218) -> (-19.685, 95.996) centre (-19.685, 93.218) ccw
  line L6 (-16.907, 93.218) -> (-16.907, 43.878)
  arc A7 (-16.907, 43.878) -> (-13.907, 40.878) centre (-13.907, 43.878) ccw
  line L7 (-13.907, 40.878) -> (-1.143, 40.878)
  arc A8 (1.127, 38.608) -> (-1.143, 40.878) centre (-1.143, 38.608) ccw
  line L8 (1.127, 38.608) -> (1.127, 1.524)
  arc A9 (-1.397, -1) -> (1.127, 1.524) centre (-1.397, 1.524) ccw
  line L9 (-1.397, -1) -> (-92.583, -1)
  arc A10 (-95.361, 1.778) -> (-92.583, -1) centre (-92.583, 1.778) ccw
  line L10 (-95.361, 1.778) -> (-95.361, 93.472)
  arc A11 (-92.837, 95.996) -> (-95.361, 93.472) centre (-92.837, 93.472) ccw
  line L11 (-92.837, 95.996) -> (-19.685, 95.996)
  arc A12 (-11.907, 93.218) -> (-19.685, 100.996) centre (-19.685, 93.218) ccw
  line L12 (-19.685, 100.996) -> (-92.837, 100.996)
  arc A13 (-92.837, 100.996) -> (-100.361, 93.472) centre (-92.837, 93.472) ccw
  line L13 (-100.361, 93.472) -> (-100.361, 1.778)
  arc A14 (-100.361, 1.778) -> (-92.583, -6) centre (-92.583, 1.778) ccw
  line L14 (-92.583, -6) -> (-1.397, -6)
  arc A15 (-1.397, -6) -> (6.127, 1.524) centre (-1.397, 1.524) ccw
  line L15 (6.127, 1.524) -> (6.127, 38.608)
  arc A16 (6.127, 38.608) -> (-1.143, 45.878) centre (-1.143, 38.608) ccw
  line L16 (-1.143, 45.878) -> (-10.907, 45.878)
  arc A17 (-11.907, 46.878) -> (-10.907, 45.878) centre (-10.907, 46.878) ccw
  line L17 (-11.907, 46.878) -> (-11.907, 93.218)
extrude "Extrude2'" cut sketch "Sketch2 (2)" against normal blind 2.5 contours A6 L6 A7 L7 A8 L8 A9 L9 A10 L10 A11 L11 bodies 3 in component "BaseLayer"
sketch "Sketch3" plane through (0, -2.5, 0) normal (0, 1, 0) x (-1, 0, 0) in component "BaseLayer"
  arc A0 (-95.361, 1.778) -> (-92.583, -1) centre (-92.583, 1.778) ccw
  line L0 (-92.583, -1) -> (-1.397, -1)
  arc A1 (-1.397, -1) -> (1.127, 1.524) centre (-1.397, 1.524) ccw
  line L1 (1.127, 1.524) -> (1.127, 38.608)
  arc A2 (1.127, 38.608) -> (-1.143, 40.878) centre (-1.143, 38.608) ccw
  line L2 (-1.143, 40.878) -> (-13.907, 40.878)
  arc A3 (-16.907, 43.878) -> (-13.907, 40.878) centre (-13.907, 43.878) ccw
  line L3 (-16.907, 43.878) -> (-16.907, 93.218)
  arc A4 (-16.907, 93.218) -> (-19.685, 95.996) centre (-19.685, 93.218) ccw
  line L4 (-19.685, 95.996) -> (-92.837, 95.996)
  arc A5 (-92.837, 95.996) -> (-95.361, 93.472) centre (-92.837, 93.472) ccw
  line L5 (-95.361, 93.472) -> (-95.361, 1.778)
  line L6 (-24.907, 87.996) -> (-87.361, 87.996)
  line L7 (-87.361, 87.996) -> (-87.361, 7)
  line L8 (-87.361, 7) -> (-6.873, 7)
  line L9 (-6.873, 7) -> (-6.873, 32.878)
  line L10 (-6.873, 32.878) -> (-13.907, 32.878)
  arc A6 (-24.907, 43.878) -> (-13.907, 32.878) centre (-13.907, 43.878) ccw
  line L11 (-24.907, 43.878) -> (-24.907, 87.996)
  circle A7 centre (-19.685, 93.496) radius 2
  circle A8 centre (-92.837, 93.496) radius 2
  circle A9 centre (-92.861, 1.778) radius 2
  circle A10 centre (-1.397, 1.5) radius 2
  circle A11 centre (-1.373, 38.378) radius 2
  line L12 (-19.685, 93.496) -> (-92.837, 93.496)
  arc A12 (-92.837, 93.496) -> (-92.861, 93.472) centre (-92.837, 93.472) ccw
  line L13 (-92.861, 93.472) -> (-92.861, 1.778)
  arc A13 (-92.861, 1.778) -> (-92.583, 1.5) centre (-92.583, 1.778) ccw
  line L14 (-92.583, 1.5) -> (-1.397, 1.5)
  arc A14 (-1.397, 1.5) -> (-1.373, 1.524) centre (-1.397, 1.524) ccw
  line L15 (-1.373, 1.524) -> (-1.373, 38.378)
  line L16 (-1.373, 38.378) -> (-13.907, 38.378)
  arc A15 (-19.407, 43.878) -> (-13.907, 38.378) centre (-13.907, 43.878) ccw
  line L17 (-19.407, 43.878) -> (-19.407, 93.218)
  arc A16 (-19.407, 93.218) -> (-19.685, 93.496) centre (-19.685, 93.218) ccw
  dimension "d34" = -2.5
  dimension "d35" = -8
  dimension "d40" = 4
  dimension "d41" = 4
  dimension "d42" = 4
  dimension "d43" = 4
  dimension "d44" = 4
  constraint coincident A7.centre L12.start
  constraint coincident A8.centre L12.end
  constraint coincident A9.centre L13.end
  constraint coincident A10.centre L14.end
  constraint coincident A11.centre L15.end
  measures "d40" diameter of A7
  measures "d41" diameter of A8
  measures "d42" diameter of A9
  measures "d43" diameter of A10
  measures "d44" diameter of A11
extrude "Extrude3" cut sketch "Sketch3" against normal through all contours L6 L7 L8 L9 L10 A6 L11 bodies 3 in component "BaseLayer"
extrude "Extrude4" cut sketch "Sketch3" against normal blind 1.5 contours A7 L12 L17 A16 | A7 L12 L17 A16 | A7 A8 A9 A10 A11 L12 L13 L14 L15 L16 A15 L17 | A8 L12 A12 L13 | A8 L12 A12 L13 | A9 L13 A13 L14 | A9 L13 A13 L14 | A11 L15 L16 | A11 L15 L16 | A10 L14 A14 L15 | A10 L14 A14 L15 bodies 3 in component "BaseLayer"
fillet "Fillet1" radius 3 5 edges at (6.873, -5, 7) (87.361, -5, 7) (6.873, -5, 32.878) (24.907, -5, 87.996) (87.361, -5, 87.996) on bodies 3 in component "BaseLayer"
sketch "Sketch3 (2)" plane through (0, 9, 0) normal (0, 1, 0) x (-1, 0, 0) in component "TopLayer"
  line L0 (-39.838, 78.573) -> (-53.888, 78.573)
  line L1 (-53.888, 78.573) -> (-53.888, 92.623)
  line L2 (-53.888, 92.623) -> (-39.838, 92.623)
  line L3 (-39.838, 92.623) -> (-39.838, 78.573)
  line L4 (-20.788, 78.573) -> (-34.838, 78.573)
  line L5 (-34.838, 78.573) -> (-34.838, 92.623)
  line L6 (-34.838, 92.623) -> (-20.788, 92.623)
  line L7 (-20.788, 92.623) -> (-20.788, 78.573)
  line L8 (-58.888, 78.573) -> (-72.938, 78.573)
  line L9 (-72.938, 78.573) -> (-72.938, 92.623)
  line L10 (-72.938, 92.623) -> (-58.888, 92.623)
  line L11 (-58.888, 92.623) -> (-58.888, 78.573)
  line L12 (-77.938, 69.048) -> (-91.988, 69.048)
  line L13 (-91.988, 69.048) -> (-91.988, 83.098)
  line L14 (-91.988, 83.098) -> (-77.938, 83.098)
  line L15 (-77.938, 83.098) -> (-77.938, 69.048)
  line L16 (-39.838, 40.473) -> (-53.888, 40.473)
  line L17 (-53.888, 40.473) -> (-53.888, 54.523)
  line L18 (-53.888, 54.523) -> (-39.838, 54.523)
  line L19 (-39.838, 54.523) -> (-39.838, 40.473)
  line L20 (-20.788, 40.473) -> (-34.838, 40.473)
  line L21 (-34.838, 40.473) -> (-34.838, 54.523)
  line L22 (-34.838, 54.523) -> (-20.788, 54.523)
  line L23 (-20.788, 54.523) -> (-20.788, 40.473)
  line L24 (-20.788, 59.523) -> (-34.838, 59.523)
  line L25 (-34.838, 59.523) -> (-34.838, 73.573)
  line L26 (-34.838, 73.573) -> (-20.788, 73.573)
  line L27 (-20.788, 73.573) -> (-20.788, 59.523)
  line L28 (-39.838, 59.523) -> (-53.888, 59.523)
  line L29 (-53.888, 59.523) -> (-53.888, 73.573)
  line L30 (-53.888, 73.573) -> (-39.838, 73.573)
  line L31 (-39.838, 73.573) -> (-39.838, 59.523)
  line L32 (-58.888, 59.523) -> (-72.938, 59.523)
  line L33 (-72.938, 59.523) -> (-72.938, 73.573)
  line L34 (-72.938, 73.573) -> (-58.888, 73.573)
  line L35 (-58.888, 73.573) -> (-58.888, 59.523)
  line L36 (-58.888, 40.473) -> (-72.938, 40.473)
  line L37 (-72.938, 40.473) -> (-72.938, 54.523)
  line L38 (-72.938, 54.523) -> (-58.888, 54.523)
  line L39 (-58.888, 54.523) -> (-58.888, 40.473)
  line L40 (-77.938, 30.948) -> (-91.988, 30.948)
  line L41 (-91.988, 30.948) -> (-91.988, 44.998)
  line L42 (-91.988, 44.998) -> (-77.938, 44.998)
  line L43 (-77.938, 44.998) -> (-77.938, 30.948)
  line L44 (-58.888, 21.423) -> (-72.938, 21.423)
  line L45 (-72.938, 21.423) -> (-72.938, 35.473)
  line L46 (-72.938, 35.473) -> (-58.888, 35.473)
  line L47 (-58.888, 35.473) -> (-58.888, 21.423)
  line L48 (-39.838, 21.423) -> (-53.888, 21.423)
  line L49 (-53.888, 21.423) -> (-53.888, 35.473)
  line L50 (-53.888, 35.473) -> (-39.838, 35.473)
  line L51 (-39.838, 35.473) -> (-39.838, 21.423)
  line L52 (-77.938, 2.373) -> (-91.988, 2.373)
  line L53 (-91.988, 2.373) -> (-91.988, 16.423)
  line L54 (-91.988, 16.423) -> (-77.938, 16.423)
  line L55 (-77.938, 16.423) -> (-77.938, 2.373)
  line L56 (-20.788, 2.373) -> (-34.838, 2.373)
  line L57 (-34.838, 2.373) -> (-34.838, 16.423)
  line L58 (-34.838, 16.423) -> (-20.788, 16.423)
  line L59 (-20.788, 16.423) -> (-20.788, 2.373)
  line L60 (-39.838, 2.373) -> (-53.888, 2.373)
  line L61 (-53.888, 2.373) -> (-53.888, 16.423)
  line L62 (-53.888, 16.423) -> (-39.838, 16.423)
  line L63 (-39.838, 16.423) -> (-39.838, 2.373)
  line L64 (-20.788, 21.423) -> (-34.838, 21.423)
  line L65 (-34.838, 21.423) -> (-34.838, 35.473)
  line L66 (-34.838, 35.473) -> (-20.788, 35.473)
  line L67 (-20.788, 35.473) -> (-20.788, 21.423)
  line L68 (-58.888, 2.373) -> (-72.938, 2.373)
  line L69 (-72.938, 2.373) -> (-72.938, 16.423)
  line L70 (-72.938, 16.423) -> (-58.888, 16.423)
  line L71 (-58.888, 16.423) -> (-58.888, 2.373)
  line L72 (-1.644, -6) -> (-1.397, -6)
  arc A0 (-1.397, -6) -> (6.127, 1.524) centre (-1.397, 1.524) ccw
  line L73 (6.127, 1.524) -> (6.127, 38.608)
  arc A1 (6.127, 38.608) -> (-1.143, 45.878) centre (-1.143, 38.608) ccw
  line L74 (-1.143, 45.878) -> (-10.907, 45.878)
  arc A2 (-11.907, 46.878) -> (-10.907, 45.878) centre (-10.907, 46.878) ccw
  line L75 (-11.907, 46.878) -> (-11.907, 93.218)
  arc A3 (-11.907, 93.218) -> (-19.685, 100.996) centre (-19.685, 93.218) ccw
  line L76 (-19.685, 100.996) -> (-92.837, 100.996)
  arc A4 (-92.837, 100.996) -> (-100.361, 93.472) centre (-92.837, 93.472) ccw
  line L77 (-100.361, 93.472) -> (-100.361, 1.778)
  arc A5 (-100.361, 1.778) -> (-92.583, -6) centre (-92.583, 1.778) ccw
  line L78 (-92.583, -6) -> (-16.644, -6)
  line L79 (-16.644, -6) -> (-16.644, -1)
  line L80 (-16.644, -1) -> (-18.661, -1)
  line L81 (-18.661, -1) -> (-18.661, 40.878)
  line L82 (-18.661, 40.878) -> (-1.143, 40.878) construction
  arc A6 (1.127, 38.608) -> (-1.143, 40.878) centre (-1.143, 38.608) ccw construction
  line L83 (1.127, 38.608) -> (1.127, 1.524) construction
  arc A7 (-1.397, -1) -> (1.127, 1.524) centre (-1.397, 1.524) ccw construction
  line L84 (-1.397, -1) -> (-1.644, -1)
  line L85 (-1.644, -1) -> (-1.644, -6)
  line L86 (-92.837, 95.996) -> (-19.685, 95.996) construction
  arc A8 (-92.837, 95.996) -> (-95.361, 93.472) centre (-92.837, 93.472) ccw construction
  line L87 (-95.361, 1.778) -> (-95.361, 93.472) construction
  arc A9 (-95.361, 1.778) -> (-92.583, -1) centre (-92.583, 1.778) ccw construction
  line L88 (-1.397, -1) -> (-92.583, -1) construction
  arc A10 (-1.397, -1) -> (1.127, 1.524) centre (-1.397, 1.524) ccw
  line L89 (1.127, 38.608) -> (1.127, 1.524)
  arc A11 (1.127, 38.608) -> (-1.143, 40.878) centre (-1.143, 38.608) ccw
  line L90 (-13.907, 40.878) -> (-1.143, 40.878)
  arc A12 (-16.907, 43.878) -> (-13.907, 40.878) centre (-13.907, 43.878) ccw construction
  line L91 (-16.907, 93.218) -> (-16.907, 43.878) construction
  arc A13 (-16.907, 93.218) -> (-19.685, 95.996) centre (-19.685, 93.218) ccw construction
  line L92 (-94.5473, -0.1863) -> (-98.0829, -3.7219) construction
  line L93 (-94.6217, 95.2567) -> (-98.1573, 98.7923) construction
  line L94 (-17.7207, 95.1823) -> (-14.1851, 98.7179) construction
  line L95 (0.4621, 40.2131) -> (3.9977, 43.7487) construction
  line L96 (0.3877, -0.2607) -> (3.9233, -3.7963) construction
  circle A14 centre (2.1555, -2.0285) radius 1.5875
  circle A15 centre (2.2299, 41.9809) radius 1.5875
  circle A16 centre (-96.3151, -1.9541) radius 1.5875
  circle A17 centre (-96.3895, 97.0245) radius 1.5875
  circle A18 centre (-15.9529, 96.9501) radius 1.5875
  dimension "d45" = 3.175
  constraint midpoint A9 L92.start
  constraint midpoint A5 L92.end
  constraint midpoint A8 L93.start
  constraint midpoint A4 L93.end
  constraint midpoint A13 L94.start
  constraint midpoint A3 L94.end
  constraint midpoint A11 L95.start
  constraint midpoint A1 L95.end
  constraint midpoint A10 L96.start
  constraint midpoint A0 L96.end
  constraint midpoint L96 A14.centre
  constraint midpoint L95 A15.centre
  constraint midpoint L92 A16.centre
  constraint midpoint L93 A17.centre
  constraint midpoint L94 A18.centre
  constraint equal A17 A18
  constraint equal A16 A18
  constraint equal A15 A16
  constraint equal A14 A15
  measures "d45" diameter of A14
extrude "Extrude2''" cut sketch "Sketch3 (2)" against normal through all contours A14 | A15 | A16 | A17 | A18 bodies 1 in component "MidLayer"
extrude "Extrude3'" cut sketch "Sketch3 (2)" against normal through all contours A14 | A15 | A16 | A17 | A18 bodies 2 in component "TopLayer"
extrude "Extrude5" cut sketch "Sketch3 (2)" against normal through all contours A14 | A15 | A16 | A17 | A18 bodies 3 in component "BaseLayer"